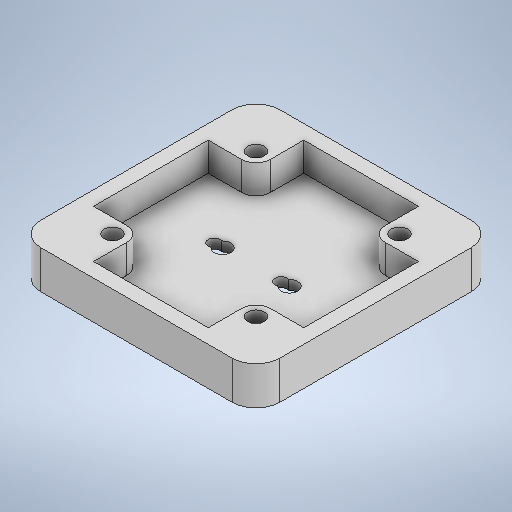
# Autodesk Inventor part: LowerCase
Saved by Autodesk Inventor 2025 (Build 290162010, 162A)
## iProperties
Created: 2025-11-03
Part Number: LowerCase
Material: Genérico
Document SubType Name: Modeling
Designer: João Vitor
Density: 1 g/cm^3
Appearance: Padrão
Author: João Vitor
Autodesk Inventor part; units mm, degrees
ref_plane "YZ Plane" through (0, 0, 0) normal (1, 0, 0) x (0, 1, 0)
ref_plane "XZ Plane" through (0, 0, 0) normal (0, 1, 0) x (-1, 0, 0)
ref_plane "XY Plane" through (0, 0, 0) normal (0, 0, 1) x (1, 0, 0)
sketch "Esboço1" plane through (0, 0, 0) normal (0, 1, 0) x (-1, 0, 0)
  line L0 (-20, 22) -> (20, 22)
  line L1 (22, 20) -> (22, -20)
  line L2 (20, -22) -> (-20, -22)
  line L3 (-22, -20) -> (-22, 20)
  line L4 (-22, 22) -> (22, -22) construction
  line L5 (22, 22) -> (-22, -22) construction
  circle A0 centre (-15, 15) radius 3
  circle A1 centre (-15, -15) radius 3
  circle A2 centre (15, -15) radius 3
  circle A3 centre (15, 15) radius 3
  circle A4 centre (-15, 15) radius 1.75
  circle A5 centre (-15, -15) radius 1.75
  circle A6 centre (15, -15) radius 1.75
  circle A7 centre (15, 15) radius 1.75
  arc A8 (22, 20) -> (20, 22) centre (20, 20) ccw
  arc A9 (20, -22) -> (22, -20) centre (20, -20) ccw
  arc A10 (-22, -20) -> (-20, -22) centre (-20, -20) ccw
  arc A11 (-20, 22) -> (-22, 20) centre (-20, 20) ccw
  line L6 (-12, 15) -> (-12, 22)
  line L7 (-15, 12) -> (-22, 12)
  line L8 (-15, -12) -> (-22, -12)
  line L9 (-12, -15) -> (-12, -22)
  line L10 (12, -15) -> (12, -22)
  line L11 (15, -12) -> (22, -12)
  line L12 (15, 12) -> (22, 12)
  line L13 (12, 15) -> (12, 22)
  line L14 (-20, 25) -> (20, 25)
  line L15 (25, 20) -> (25, -20)
  line L16 (20, -25) -> (-20, -25)
  line L17 (-25, -20) -> (-25, 20)
  line L18 (-25, 25) -> (25, -25) construction
  line L19 (25, 25) -> (-25, -25) construction
  arc A12 (-25, -20) -> (-20, -25) centre (-20, -20) ccw
  arc A13 (-20, 25) -> (-25, 20) centre (-20, 20) ccw
  arc A14 (25, 20) -> (20, 25) centre (20, 20) ccw
  arc A15 (20, -25) -> (25, -20) centre (20, -20) ccw
  circle A16 centre (7, 0) radius 1.75
  circle A17 centre (-7, 0) radius 1.75
  circle A18 centre (8.75, 0) radius 1.25
  circle A19 centre (-5.25, 0) radius 1.25
  point P0 (0, 0)
  point P1 (8.3036, 1.1676)
  point P2 (8.3036, -1.1676)
  point P3 (-5.6964, 1.1676)
  point P4 (-5.6964, -1.1676)
  dimension "d18" = 3.5
  dimension "d19" = 3.5
  dimension "d0" = 44
  dimension "d1" = 44
  dimension "d2" = 6
  dimension "d3" = 7
  dimension "d4" = 7
  dimension "d7" = 3.5
  dimension "d8" = 2
  dimension "d9" = 3
  dimension "d10" = 3
  dimension "d11" = 5
  dimension "d20" = 2.5
  dimension "d21" = 2.5
  dimension "d22" = 7
  dimension "d23" = 7
  constraints: 40 end point, 32 point on line, 24 point on circle, 23 tangent, 18 centre point, 12 equal radius, 7 perpendicular, 6 horizontal alignment, 5 parallel, 4 midpoint, 3 concentric, 3 horizontal, 1 coincident, 1 vertical alignment, 6 other
  measures "d0" distance of L5.start L4.end
  measures "d1" distance of L4.end L5.end
  measures "d2" diameter of A3
  measures "d3" distance from line of L3 A0.centre
  measures "d4" distance from line of L0 A0.centre
  measures "d7" diameter of A4
  measures "d8" radius of A8
  measures "d9" distance between parallel lines of L0 L14
  measures "d10" distance between parallel lines of L15 L1
  measures "d11" radius of A12
  measures "d20" diameter of A18
  measures "d21" diameter of A19
  measures "d22" distance of point (-7, 0) point (0, 0)
  measures "d23" distance of point (7, 0) point (0, 0)
extrude "Extrusão1" add sketch "Esboço1" along normal blind 2 contours L0 L13 A3 L12 L1 L11 A2 L10 L2 L9 A1 L8 L3 L7 A0 L6 | A16 A18 | A16 A18 | A18 A16 | A17 A19 | A17 A19 | A19 A17
extrude "Extrusão2" add sketch "Esboço1" along normal blind 8 contours L0 L6 A0 L7 L3 A11 | L0 A8 L1 L12 A3 L13 | A0 | A3 | L8 A1 L9 L2 A10 L3 | A1 | L1 A9 L2 L10 A2 L11 | A2
extrude "Extrusão3" add sketch "Esboço1" along normal blind 8 contours L14 A14 L15 A15 L16 A12 L17 A13
extrude "Extrusão4" cut sketch "Esboço1" along normal blind 3.5 contours A16 A18 | A16 A18 | A18 A16 | A17 A19 | A17 A19 | A19 A17
extrude "Extrusão5" cut sketch "Esboço1" along normal blind 2 contours A0 | A3 | A1 | A2 | A4 | A5 | A6 | A7
equation "\"d24\" = d18"
